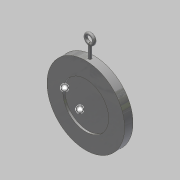
# Autodesk Inventor part: CHECK VALVE SWING WAFER 304L DN65
Saved by Autodesk Inventor 2017 (Build 210142000, 142)
## iProperties
Created: 2015-03-19
Part Number: CHECK VALVE SWING WAFER 304L DN65
Material: 304L
Document SubType Name: Modeling
Designer: m_crauwels
Density: 8 g/cm^3
Appearance: Steel
Mass: 365.342 g
Surface Area: 480.363 cm^2
Volume: 45.6678 cm^3
Description: BV38-6666E-PN10/PN16
Catalog Web Link: http://www.pocketbrewery.com
PipeDiameter: 76.100 mm
DiamExt: 129.000 mm
Thickness: 14.000 mm
Author: m_crauwels
Autodesk Inventor part; units mm, degrees
ref_plane "YZ Plane" through (0, 0, 0) normal (1, 0, 0) x (0, 1, 0)
ref_plane "XZ Plane" through (0, 0, 0) normal (0, 1, 0) x (-1, 0, 0)
ref_plane "XY Plane" through (0, 0, 0) normal (0, 0, 1) x (1, 0, 0)
sketch "Sketch1" plane through (0, 0, 0) normal (0, 1, 0) x (-1, 0, 0)
  line L0 (7, 0) -> (-7, 0) construction
  line L1 (7, 64.5) -> (-7, 64.5)
  line L2 (-7, 64.5) -> (-7, 38.05)
  line L3 (7, 38.05) -> (-7, 38.05)
  line L4 (7, 38.05) -> (7, 64.5)
  line L5 (3.5, 0) -> (-3.5, 0)
  line L6 (-3.5, 0) -> (-3.5, 38.05)
  line L7 (-3.5, 38.05) -> (3.5, 38.05)
  line L8 (3.5, 38.05) -> (3.5, 0)
  line L9 (3.5, 0) -> (-3.5, 38.05) construction
  line L10 (-3.5, 0) -> (3.5, 38.05) construction
  point P0 (0, 19.025)
  point P1 (0, 38.05)
  point P2 (0, 0)
  point P3 (0, 0)
  dimension "Thickness" = 14
  dimension "DiamExt" = 129
  dimension "PipeDiameter" = 76.1
  dimension "d8" = 7
  constraints: 22 end point, 6 midpoint, 4 perpendicular, 2 horizontal, 2 parallel, 1 coincident, 1 point on line
  measures "Thickness" distance of L1.start L1.end
  measures "DiamExt" diameter of L1 L0
  measures "PipeDiameter" diameter of L3 L0
  measures "d8" distance of L6.end L7.end
revolve "Revolution1" add sketch "Sketch1" angle 360 about axis through (-7, 0, 0) along (1, 0, 0)
sketch "Sketch3" plane through (0, 0, 0) normal (0, 0, 1) x (1, 0, 0)
  circle A0 centre (0, 0) radius 2.5
  dimension "d9" = 5
  constraints: 1 centre point, 1 coincident
  measures "d9" diameter of A0
sketch "Sketch4" plane through (0, 0, 0) normal (1, 0, 0) x (0, 1, 0)
  line L0 (0, 0) -> (0, 85.5)
  arc A0 (0, 85.5) -> (-0.9974, 85.5714) centre (0, 92.5) ccw
  dimension "d10" = 7
  dimension "d11" = 92.5
  dimension "d14" = 1
  constraints: 2 end point, 2 point on circle, 1 centre point, 1 point on line, 1 vertical
  measures "d10" radius of A0
  measures "d11" distance of A0.centre L0.start
  measures "d14" distance of A0.end L0.end
sweep "Sweep1" add profiles "Sketch3" path "Sketch4"
equation "\"d8\" = 0.5 * Thickness"
equation "\"d10\" = 0.5 * Thickness"
equation "\"d11\" = 0.5 * DiamExt + 2 * Thickness"
body "Solid1"
